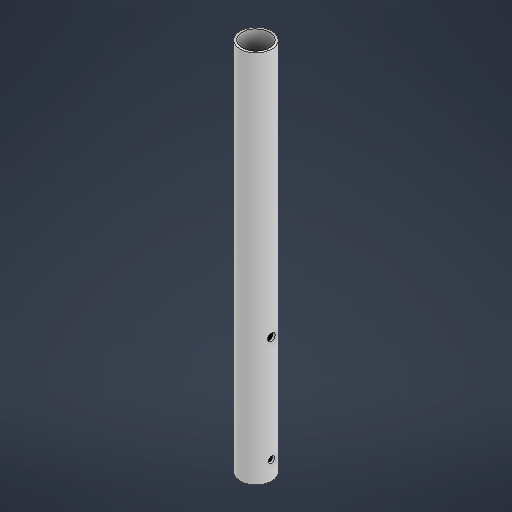
# Autodesk Inventor part: stickshift
Saved by Autodesk Inventor 2026.2 (Build 302298010, 298A)
## iProperties
Created: 2026-07-07
Part Number: stickshift
Material: Generic
Document SubType Name: Modeling
Designer: tasle
Density: 1 g/cm^3
Appearance: Default
Author: tasle
Autodesk Inventor part; units mm, degrees
ref_plane "YZ Plane" through (0, 0, 0) normal (1, 0, 0) x (0, 1, 0)
ref_plane "XZ Plane" through (0, 0, 0) normal (0, 1, 0) x (-1, 0, 0)
ref_plane "XY Plane" through (0, 0, 0) normal (0, 0, 1) x (1, 0, 0)
sketch "Sketch1" plane through (0, 0, 0) normal (0, 1, 0) x (-1, 0, 0)
  circle A0 centre (0, 0) radius 12.7
  circle A1 centre (0, 0) radius 11
  dimension "d0" = 25.4
  dimension "d1" = 22
  constraints: 2 centre point, 2 coincident
  measures "d0" diameter of A0
  measures "d1" diameter of A1
extrude "Extrusion1" add sketch "Sketch1" along normal blind 300
sketch "Sketch2" plane through (0, 0, 0) normal (1, 0, 0) x (0, 1, 0)
  circle A0 centre (100, 0) radius 3
  line L0 (0, -12.7) -> (0, 12.7) projected
  circle A1 centre (15, 0) radius 2.5
  point P0 (0, 0)
  dimension "d4" = 6
  dimension "d5" = 100
  dimension "d6" = 5
  dimension "d7" = 15
  constraints: 2 centre point
  measures "d4" diameter of A0
  measures "d5" distance from line of L0 A0.centre
  measures "d6" diameter of A1
  measures "d7" distance from line of L0 A1.centre
extrude "Extrusion2" cut sketch "Sketch2" along normal mid plane 300
body "Solid1"
